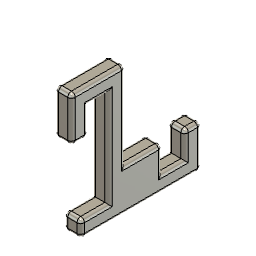
Project hooks v1 (Autodesk Fusion 360 design; units mm, degrees)
Autodesk Fusion 360 part; units mm, degrees
sketch "Sketch1" plane through (0, 0, 0) normal (1, 0, 0) x (0, 0, -1)
  line L0 (-50, 20) -> (-4, 20)
  line L1 (-4, 20) -> (-4, -11.5)
  line L2 (-4, -11.5) -> (-50, -11.5)
  line L3 (-50, -11.5) -> (-50, 20)
  line L4 (-65.5096, 6.4803) -> (-1.0096, 6.4803)
  line L5 (-1.0096, 6.4803) -> (-1.0096, -9.308)
  line L6 (-1.0096, -9.308) -> (-65.5096, -9.308)
  line L7 (-65.5096, -9.308) -> (-65.5096, 6.4803)
  line L8 (52, 50) -> (64.5, 50)
  line L9 (65.5, 49) -> (65.5, 45.5)
  line L10 (65.5, 45.5) -> (51, 45.5)
  line L11 (51, 45.5) -> (51, 49)
  line L12 (51, 45.5) -> (55.5, 45.5)
  line L13 (55.5, 45.5) -> (55.5, 39)
  line L14 (54.5, 38) -> (52, 38)
  line L15 (51, 39) -> (51, 45.5)
  line L16 (65.5, 45.5) -> (61, 45.5)
  line L17 (61, 45.5) -> (61, 19.5)
  line L18 (61, 19.5) -> (65.5, 19.5)
  line L19 (65.5, 19.5) -> (65.5, 45.5)
  line L20 (65.5, 19.5) -> (54.5, 19.5)
  line L21 (53.5, 18.5) -> (53.5, 16)
  line L22 (54.5, 15) -> (65.5, 15)
  line L23 (65.5, 15) -> (65.5, 19.5)
  line L24 (65.5, 15) -> (75.5, 15)
  line L25 (75.5, 15) -> (75.5, 25.5)
  line L26 (74.5, 26.5) -> (65.5, 26.5)
  line L27 (65.5, 26.5) -> (65.5, 15)
  line L28 (75.5, 15) -> (85, 15)
  line L29 (86, 16) -> (86, 19.5)
  line L30 (86, 19.5) -> (75.5, 19.5)
  line L31 (75.5, 19.5) -> (75.5, 15)
  line L32 (86, 19.5) -> (81.5, 19.5)
  line L33 (81.5, 19.5) -> (81.5, 25.5)
  line L34 (82.5, 26.5) -> (85, 26.5)
  line L35 (86, 25.5) -> (86, 19.5)
  arc A0 (52, 50) -> (51, 49) centre (52, 49) ccw
  arc A1 (65.5, 49) -> (64.5, 50) centre (64.5, 49) ccw
  arc A2 (51, 39) -> (52, 38) centre (52, 39) ccw
  arc A3 (54.5, 38) -> (55.5, 39) centre (54.5, 39) ccw
  arc A4 (54.5, 19.5) -> (53.5, 18.5) centre (54.5, 18.5) ccw
  arc A5 (53.5, 16) -> (54.5, 15) centre (54.5, 16) ccw
  arc A6 (75.5, 25.5) -> (74.5, 26.5) centre (74.5, 25.5) ccw
  arc A7 (82.5, 26.5) -> (81.5, 25.5) centre (82.5, 25.5) ccw
  arc A8 (86, 25.5) -> (85, 26.5) centre (85, 25.5) ccw
  arc A9 (85, 15) -> (86, 16) centre (85, 16) ccw
  point P0 (51, 50)
  point P1 (65.5, 50)
  point P2 (51, 38)
  point P3 (53.5, 19.5)
  point P4 (86, 15)
  point P5 (86, 26.5)
  dimension "d1" = 46
  dimension "d2" = 31.5
  dimension "d3" = 64.5
  dimension "d4" = 14.5
  dimension "d5" = 4.5
  dimension "d6" = 4.5
  dimension "d7" = 7.5
  dimension "d8" = 4.5
  dimension "d9" = 26
  dimension "d10" = 12
  dimension "d11" = 4.5
  dimension "d12" = 10
  dimension "d13" = 11.5
  dimension "d14" = 10.5
  dimension "d15" = 4.5
  dimension "d16" = 4.5
  dimension "d17" = 7
  dimension "d18" = 1
  constraint horizontal L0
  constraint vertical L1
  constraint horizontal L2
  constraint vertical L3
  constraint horizontal L4
  constraint vertical L5
  constraint horizontal L6
  constraint vertical L7
  constraint horizontal L8
  constraint vertical L9
  constraint horizontal L10
  constraint vertical L11
  constraint horizontal L12
  constraint vertical L13
  constraint horizontal L14
  constraint vertical L15
  constraint horizontal L16
  constraint vertical L17
  constraint horizontal L18
  constraint vertical L19
  constraint horizontal L20
  constraint vertical L21
  constraint horizontal L22
  constraint vertical L23
  constraint horizontal L24
  constraint vertical L25
  constraint horizontal L26
  constraint vertical L27
  constraint horizontal L28
  constraint vertical L29
  constraint horizontal L30
  constraint vertical L31
  constraint horizontal L32
  constraint vertical L33
  constraint horizontal L34
  constraint vertical L35
  constraint coincident P0 L8
  constraint coincident P0 L11
  constraint tangent L8 A0
  constraint tangent L11 A0
  constraint coincident P1 L8
  constraint coincident P1 L9
  constraint tangent L8 A1
  constraint tangent L9 A1
  constraint equal A0 A1
  constraint coincident P2 L14
  constraint coincident P2 L15
  constraint tangent L14 A2
  constraint tangent L15 A2
  constraint equal A0 A2
  constraint tangent L13 A3
  constraint tangent L14 A3
  constraint equal A0 A3
  constraint coincident P3 L20
  constraint coincident P3 L21
  constraint tangent L20 A4
  constraint tangent L21 A4
  constraint equal A0 A4
  constraint tangent L21 A5
  constraint tangent L22 A5
  constraint equal A0 A5
  constraint tangent L25 A6
  constraint tangent L26 A6
  constraint equal A0 A6
  constraint tangent L33 A7
  constraint tangent L34 A7
  constraint equal A0 A7
  constraint coincident P5 L34
  constraint coincident P5 L35
  constraint tangent L34 A8
  constraint tangent L35 A8
  constraint equal A0 A8
  constraint coincident P4 L28
  constraint coincident P4 L29
  constraint tangent L28 A9
  constraint tangent L29 A9
  constraint equal A0 A9
  measures "d1" distance of L0.start L0.end
  measures "d2" distance of L0.start L2.end
  measures "d3" distance of L4.start L4.end
  measures "d4" distance of P0 P1
  measures "d5" distance of P0 L10.end
  measures "d6" distance of L10.end L12.end
  measures "d7" distance of L10.end P2
  measures "d8" distance of L9.end L16.end
  measures "d9" distance of L9.end L18.end
  measures "d10" distance of L18.end P3
  measures "d11" distance of L18.end L22.end
  measures "d12" distance of L22.end L24.end
  measures "d13" distance of L22.end L26.end
  measures "d14" distance of L24.end P4
  measures "d15" distance of L24.end L30.end
  measures "d16" distance of L29.end L32.end
  measures "d17" distance of L29.end P5
  measures "d18" radius of A0
extrude "Extrude1" add sketch "Sketch1" along normal blind 4.5 contours L8 L9 L10 L11 L12 L16 A0 A1 | L10 L12 L13 L14 L15 A2 A3 | L10 L16 L17 L18 L19 L20 L27 | L19 L23 L24 L25 L26 L27 L31 A6 | L18 L20 L21 L22 L23 L27 A4 A5 | L25 L28 L29 L30 L31 L32 A9 | L30 L32 L33 L34 L35 A7 A8
fillet "Fillet1" radius 1 26 edges at (4.5, 37.75, -65.5) (4.5, 49.7071, -65.2071) (4.5, 50, -58.25) (4.5, 49.7071, -51.2929) (4.5, 44, -51) (4.5, 38.2929, -51.2929) (4.5, 38, -53.25) (4.5, 38.2929, -55.2071) (4.5, 42.25, -55.5) (4.5, 22.5, -75.5) (4.5, 26.2071, -75.2071) (4.5, 26.5, -70) (4.5, 19.5, -78.5) (4.5, 19.5, -57.75) (4.5, 19.2071, -53.7929) (4.5, 17.25, -53.5) (4.5, 15.2929, -53.7929) (4.5, 15, -69.75) (4.5, 15.2929, -85.7071) (4.5, 20.75, -86) (4.5, 26.2071, -85.7071) (4.5, 26.5, -83.75) (4.5, 26.2071, -81.7929) (4.5, 22.5, -81.5) (4.5, 32.5, -61) (4.5, 45.5, -58.25)
fillet "Fillet2" radius 1 26 edges at (0, 22.5, -75.5) (0, 26.2071, -75.2071) (0, 26.5, -70) (0, 37.75, -65.5) (0, 49.7071, -65.2071) (0, 50, -58.25) (0, 49.7071, -51.2929) (0, 44, -51) (0, 38.2929, -51.2929) (0, 38, -53.25) (0, 38.2929, -55.2071) (0, 42.25, -55.5) (0, 45.5, -58.25) (0, 32.5, -61) (0, 19.5, -57.75) (0, 19.2071, -53.7929) (0, 17.25, -53.5) (0, 15.2929, -53.7929) (0, 15, -69.75) (0, 15.2929, -85.7071) (0, 20.75, -86) (0, 26.2071, -85.7071) (0, 26.5, -83.75) (0, 26.2071, -81.7929) (0, 22.5, -81.5) (0, 19.5, -78.5)
equation "d4 = 4.5 mm + 5.5 mm + 4.5 mm"
equation "d7 = 12 mm - d5"
equation "d10 = 4.5 mm + 7.5 mm"
equation "d12 = 5.5 mm + 4.5 mm"
equation "d13 = 4.5 mm + 7 mm"
equation "d14 = 6 mm + 4.5 mm"
